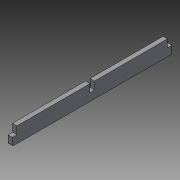
# Autodesk Inventor part: comb_spacer
Saved by Autodesk Inventor 2014 SP1 (Build 180222100, 222)
## iProperties
Created: 2014-11-11
Part Number: comb_spacer
Material: Generic
Document SubType Name: Modeling
Designer: rawrdong
Density: 1 g/cm^3
Appearance: Default
Author: rawrdong
Autodesk Inventor part; units mm, degrees
ref_plane "YZ Plane" through (0, 0, 0) normal (1, 0, 0) x (0, 1, 0)
ref_plane "XZ Plane" through (0, 0, 0) normal (0, 1, 0) x (-1, 0, 0)
ref_plane "XY Plane" through (0, 0, 0) normal (0, 0, 1) x (1, 0, 0)
sketch "Sketch1" plane through (0, 0, 0) normal (1, 0, 0) x (0, 1, 0)
  line L0 (0, 0) -> (102.9, 0)
  line L1 (102.9, 0) -> (102.9, 10)
  line L2 (102.9, 10) -> (0, 10)
  line L3 (0, 10) -> (0, 0)
  line L4 (50, 10) -> (52.9, 10)
  line L5 (52.9, 10) -> (52.9, 5)
  line L6 (52.9, 5) -> (50, 5)
  line L7 (50, 5) -> (50, 10)
  line L8 (102.9, 10) -> (100, 10)
  line L9 (100, 10) -> (100, 5)
  line L10 (100, 5) -> (102.9, 5)
  line L11 (102.9, 5) -> (102.9, 10)
  line L12 (2.9, 5) -> (0, 5)
  line L13 (0, 5) -> (0, 10)
  line L14 (0, 10) -> (2.9, 10)
  line L15 (2.9, 10) -> (2.9, 5)
  line L16 (51.45, 5) -> (51.45, 0)
  point P0 (51.45, 10)
  dimension "d0" = 2.9
  dimension "d1" = 5
  dimension "d2" = 10
  dimension "d3" = 50
  constraints: 34 end point, 8 parallel, 4 collinear, 4 horizontal, 4 perpendicular, 3 midpoint, 1 coincident, 1 point on line, 1 other
  measures "d0" distance of L9.end L10.end
  measures "d1" distance of L8.end L9.end
  measures "d2" distance of L2.end L0.start
  measures "d3" distance between parallel lines of L7 L3
extrude "Extrusion1" add sketch "Sketch1" along normal blind 2.85 contours L3 L12 L15 L2 L7 L6 L16 L0 | L16 L6 L5 L2 L9 L10 L1 L0
fillet "Fillet1" radius 0.5 2 edges at (1.425, 0, 0) (1.425, 102.9, 0)
body "Solid1"
